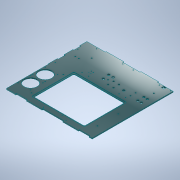
# Autodesk Inventor part: Lateral Derecho Carcasa
Saved by Autodesk Inventor 2020 (Build 240168000, 168)
## iProperties
Created: 2020-06-08
Part Number: Lateral Derecho Carcasa
Material: MDF Tablero de fibras de densidad media
Document SubType Name: Modeling
Designer: Pipi
Density: 0.8 g/cm^3
Appearance: Azul - Pintura mural - Brillante
Mass: 1380.71 g
Surface Area: 4227.94 cm^2
Volume: 1725.88 cm^3
Author: Pipi
Autodesk Inventor part; units mm, degrees
ref_plane "YZ Plane" through (0, 0, 0) normal (1, 0, 0) x (0, 1, 0)
ref_plane "XZ Plane" through (0, 0, 0) normal (0, 1, 0) x (-1, 0, 0)
ref_plane "XY Plane" through (0, 0, 0) normal (0, 0, 1) x (1, 0, 0)
sketch "Boceto1" plane through (0, 0, 0) normal (0, 1, 0) x (-1, 0, 0)
  line L0 (31.3028, -81.5323) -> (31.3028, -546.5323)
  line L1 (526.8028, -376.5323) -> (521.3028, -376.5323)
  line L2 (116.3028, -128.5323) -> (116.3028, -344.5323)
  line L3 (398.303, -351.5323) -> (123.3028, -351.5323)
  line L4 (123.3028, -121.5323) -> (399.3028, -121.5323)
  line L5 (526.8028, -376.5323) -> (526.8028, -326.5323)
  line L6 (521.3028, -416.5323) -> (521.3028, -376.5323)
  line L7 (406.3028, -344.5323) -> (406.3028, -128.5323)
  line L8 (399.3028, -351.5323) -> (123.3028, -351.5323)
  line L9 (123.3028, -121.5323) -> (399.3028, -121.5323)
  arc A0 (399.3028, -351.5323) -> (406.3028, -344.5323) centre (399.3028, -344.5323) ccw
  arc A1 (406.3028, -128.5323) -> (399.3028, -121.5323) centre (399.3028, -128.5323) ccw
  arc A2 (123.3028, -121.5323) -> (116.3028, -128.5323) centre (123.3028, -128.5323) ccw
  arc A3 (116.3028, -344.5323) -> (123.3028, -351.5323) centre (123.3028, -344.5323) ccw
  line L10 (123.3028, -114.5323) -> (399.3028, -114.5323)
  line L11 (413.3028, -128.5323) -> (413.3028, -344.5323)
  line L12 (399.3028, -358.5323) -> (123.3028, -358.5323)
  line L13 (109.3028, -344.5323) -> (109.3028, -128.5323)
  line L14 (109.3028, -128.5323) -> (109.3028, -121.5323)
  line L15 (116.3028, -114.5323) -> (123.3028, -114.5323)
  line L16 (109.3028, -344.5323) -> (109.3028, -351.5323)
  line L17 (116.3028, -358.5323) -> (123.3028, -358.5323)
  line L18 (413.3028, -344.5323) -> (413.3028, -351.5323)
  line L19 (406.3028, -358.5323) -> (399.3028, -358.5323)
  line L20 (413.3028, -128.5323) -> (413.3028, -121.5323)
  line L21 (399.3028, -114.5323) -> (406.3028, -114.5323)
  arc A4 (413.3028, -121.5323) -> (406.3028, -114.5323) centre (406.3028, -121.5323) ccw
  arc A5 (406.3028, -358.5323) -> (413.3028, -351.5323) centre (406.3028, -351.5323) ccw
  arc A6 (109.3028, -351.5323) -> (116.3028, -358.5323) centre (116.3028, -351.5323) ccw
  arc A7 (116.3028, -114.5323) -> (109.3028, -121.5323) centre (116.3028, -121.5323) ccw
  line L22 (421.3028, -552.0323) -> (421.3028, -546.5323)
  line L23 (421.3028, -546.5323) -> (521.3028, -546.5323)
  line L24 (421.3028, -552.0323) -> (321.3028, -552.0323)
  line L25 (321.3028, -552.0323) -> (321.3028, -546.5323)
  line L26 (321.3028, -546.5323) -> (221.3028, -546.5323)
  line L27 (221.3028, -546.5323) -> (221.3028, -552.0323)
  line L28 (319.3028, -81.5323) -> (319.3028, -87.0323)
  line L29 (199.3028, -81.5323) -> (199.3028, -87.0323)
  line L30 (319.3028, -87.0323) -> (199.3028, -87.0323)
  circle A8 centre (76.3028, -156.5323) radius 3
  circle A9 centre (76.3028, -276.5323) radius 3
  line L31 (31.3028, -81.5323) -> (49.3028, -81.5323)
  circle A10 centre (76.3028, -481.0323) radius 3
  line L32 (521.3028, -81.5323) -> (523.8028, -81.5323)
  line L33 (221.3028, -552.0323) -> (121.3028, -552.0323)
  line L34 (121.3028, -552.0323) -> (121.3028, -546.5323)
  line L35 (121.3028, -546.5323) -> (31.3028, -546.5323)
  line L36 (526.8028, -416.5323) -> (521.3028, -416.5323)
  line L37 (526.8028, -416.5323) -> (526.8028, -466.5323)
  line L38 (526.8028, -466.5323) -> (521.3028, -466.5323)
  line L39 (521.3028, -466.5323) -> (521.3028, -506.5323)
  line L40 (521.3028, -506.5323) -> (526.8028, -506.5323)
  line L41 (526.8028, -546.5323) -> (526.8028, -506.5323)
  circle A11 centre (41.0178, -541.5323) radius 2
  circle A12 centre (349.1778, -378.6573) radius 2
  circle A13 centre (386.4278, -378.6573) radius 2
  circle A14 centre (367.8028, -383.8623) radius 2
  line L42 (261.3028, -358.5323) -> (261.3028, -396.5323)
  circle A15 centre (173.4278, -378.6573) radius 2
  circle A16 centre (136.1778, -378.6573) radius 2
  line L43 (521.3028, -546.5323) -> (526.8028, -546.5323)
  circle A17 centre (194.3028, -94.7473) radius 2
  circle A18 centre (324.3028, -94.7473) radius 2
  circle A19 centre (461.8028, -538.0323) radius 2
  circle A20 centre (311.8028, -538.0323) radius 2
  circle A21 centre (101.3028, -538.0323) radius 2
  circle A22 centre (251.3028, -538.0323) radius 2
  circle A23 centre (513.5878, -481.5323) radius 2
  circle A24 centre (513.5878, -351.5323) radius 2
  line L44 (319.3028, -81.5323) -> (409.3028, -81.5323)
  line L45 (409.3028, -81.5323) -> (409.3028, -87.0323)
  line L46 (409.3028, -87.0323) -> (469.3028, -87.0323)
  line L47 (469.3028, -87.0323) -> (469.3028, -81.5323)
  line L48 (521.3028, -81.5323) -> (469.3028, -81.5323)
  line L49 (409.3028, -81.5323) -> (319.3028, -81.5323)
  line L50 (199.3028, -81.5323) -> (109.3028, -81.5323)
  line L51 (109.3028, -81.5323) -> (109.3028, -87.0323)
  line L52 (109.3028, -87.0323) -> (49.3028, -87.0323)
  line L53 (49.3028, -87.0323) -> (49.3028, -81.5323)
  line L54 (31.3028, -81.5323) -> (49.3028, -81.5323)
  line L55 (109.3028, -81.5323) -> (199.3028, -81.5323)
  circle A25 centre (354.4278, -397.5323) radius 1.5
  circle A26 centre (366.4278, -397.5323) radius 1.5
  line L56 (82.3528, -532.0323) -> (70.2528, -532.0323)
  line L57 (70.2528, -532.0323) -> (70.2528, -542.7823)
  line L58 (70.2528, -542.7823) -> (82.3528, -542.7823)
  line L59 (82.3528, -542.7823) -> (82.3528, -532.0323)
  line L60 (69.2528, -543.7823) -> (69.2528, -531.0323)
  line L61 (69.2528, -531.0323) -> (83.3528, -531.0323)
  line L62 (83.3528, -531.0323) -> (83.3528, -543.7823)
  line L63 (83.3528, -543.7823) -> (69.2528, -543.7823)
  circle A27 centre (518.3028, -143.5323) radius 2.25
  circle A28 centre (447.3028, -143.5323) radius 2.25
  circle A29 centre (447.3028, -298.5323) radius 2.25
  circle A30 centre (518.3028, -298.5323) radius 2.25
  circle A31 centre (518.3028, -214.5323) radius 2.25
  circle A32 centre (518.3028, -227.5323) radius 2.25
  circle A33 centre (447.3028, -214.5323) radius 2.25
  circle A34 centre (447.3028, -227.5323) radius 2.25
  circle A35 centre (482.8028, -179.0323) radius 37.5
  circle A36 centre (482.8028, -263.0323) radius 37.5
  line L64 (523.8028, -81.5323) -> (524.4028, -81.5323)
  line L65 (524.4028, -81.5323) -> (524.4028, -326.5323)
  line L66 (524.4028, -326.5323) -> (526.8028, -326.5323)
  circle A37 centre (484.8028, -438.5323) radius 3
  circle A38 centre (464.8028, -438.5323) radius 3
  circle A39 centre (366.4278, -411.5323) radius 2
  circle A40 centre (354.4278, -411.5323) radius 2
  circle A41 centre (228.4028, -106.5323) radius 2
  point P0 (0, 0)
  point P1 (398.3028, -355.6989)
  point P2 (109.3028, -358.5323)
  point P3 (413.3028, -358.5323)
  point P4 (413.3028, -114.5323)
  point P5 (398.303, -351.5323)
  dimension "d142" = 230
  dimension "d146" = 85
  dimension "d155" = 5.5
  dimension "d159" = 40
  dimension "d160" = 50
  dimension "d185" = 90
  dimension "d207" = 7
  dimension "d208" = 290
  dimension "d219" = 7
  dimension "d220" = 7
  dimension "d221" = 7
  dimension "d223" = 7
  dimension "d230" = 5.5
  dimension "d235" = 100
  dimension "d236" = 100
  dimension "d237" = 100
  dimension "d257" = 202
  dimension "d258" = 5.5
  dimension "d259" = 168
  dimension "d261" = 120
  dimension "d279" = 6
  dimension "d280" = 6
  dimension "d289" = 120
  dimension "d292" = 6
  dimension "d298" = 7
  dimension "d299" = 27.5
  dimension "d303" = 5.5
  dimension "d304" = 100
  dimension "d305" = 5.5
  dimension "d311" = 5.5
  dimension "d314" = 50
  dimension "d315" = 40
  dimension "d316" = 5.5
  dimension "d323" = 4
  dimension "d324" = 9.715
  dimension "d325" = 5
  dimension "d328" = 4
  dimension "d329" = 4
  dimension "d330" = 4
  dimension "d338" = 20.125
  dimension "d339" = 25.33
  dimension "d340" = 20.125
  dimension "d341" = 26.875
  dimension "d355" = 4
  dimension "d356" = 163
  dimension "d357" = 4
  dimension "d358" = 130
  dimension "d361" = 4
  dimension "d362" = 8.5
  dimension "d363" = 65
  dimension "d364" = 4
  dimension "d365" = 150
  dimension "d366" = 4
  dimension "d367" = 8.5
  dimension "d368" = 70
  dimension "d369" = 4
  dimension "d370" = 150
  dimension "d371" = 4
  dimension "d372" = 65
  dimension "d373" = 7.715
  dimension "d374" = 4
  dimension "d375" = 7.715
  dimension "d376" = 130
  dimension "d377" = 7.715
  constraints: 134 end point, 42 centre point, 27 perpendicular, 16 point on circle, 16 tangent, 12 horizontal, 10 point on line, 9 vertical, 6 equal radius, 5 parallel, 2 symmetric about line, 1 midpoint, 5 other
  measures "d142" distance between parallel lines of L3 L4
  measures "d146" distance between parallel lines of L0 L2
  measures "d155" distance between parallel lines of L6 L5
  measures "d159" distance of L6.start L1.end
  measures "d160" distance of L1.start L5.end
  measures "d185" angle of L1 L5
  measures "d207" radius of A0
  measures "d208" distance between parallel lines of L2 L7
  measures "d219" distance between parallel lines of L7 L11
  measures "d220" distance between parallel lines of L2 L13
  measures "d221" radius of A4
  measures "d223" distance between parallel lines of L3 L12
  measures "d230" distance of L22.start L22.end
  measures "d235" distance of L22.end L23.end
  measures "d236" distance of L22.start L24.end
  measures "d237" distance of L25.end L26.end
  measures "d257" distance of L32.start L28.start
  measures "d258" distance of L28.start L28.end
  measures "d259" distance of L0.start L29.start
  measures "d261" distance of L28.end L29.end
  measures "d279" diameter of A8
  measures "d280" diameter of A9
  measures "d289" distance of A8.centre A9.centre
  measures "d292" diameter of A10
  measures "d298" distance between parallel lines of L10 L4
  measures "d299" distance between parallel lines of L30 L10
  measures "d303" distance of L41.start L23.end
  measures "d304" distance of L27.end L33.end
  measures "d305" distance of L26.end L27.end
  measures "d311" distance of L33.end L34.end
  measures "d314" distance of L36.start L37.end
  measures "d315" distance of L38.end L39.end
  measures "d316" distance of L39.end L40.end
  measures "d323" diameter of A11
  measures "d324" distance from line of L0 A11.centre
  measures "d325" distance from line of L35 A11.centre
  measures "d328" diameter of A12
  measures "d329" diameter of A13
  measures "d330" diameter of A14
  measures "d338" distance from line of L12 A13.centre
  measures "d339" distance from line of L12 A14.centre
  measures "d340" distance from line of L12 A12.centre
  measures "d341" distance from line of L18 A13.centre
  measures "d355" diameter of A17
  measures "d356" distance from line of L0 A17.centre
  measures "d357" diameter of A18
  measures "d358" distance of A17.centre A18.centre
  measures "d361" diameter of A19
  measures "d362" distance from line of L23 A19.centre
  measures "d363" distance from line of L41 A19.centre
  measures "d364" diameter of A20
  measures "d365" distance of A20.centre A19.centre
  measures "d366" diameter of A21
  measures "d367" distance from line of L35 A21.centre
  measures "d368" distance from line of L0 A21.centre
  measures "d369" diameter of A22
  measures "d370" distance of A21.centre A22.centre
  measures "d371" diameter of A23
  measures "d372" distance from line of L23 A23.centre
  measures "d373" distance from line of L39 A23.centre
  measures "d374" diameter of A24
  measures "d375" distance from line of L6 A24.centre
  measures "d376" distance of A23.centre A24.centre
  measures "d377" distance from line of A18.centre L30
extrude "Extrusión1" add sketch "Boceto1" along normal blind 5.5 contours L31 L53 L52 L51 L50 L29 L30 L28 L44 L45 L46 L47 L48 L32 L64 L65 L66 L5 L1 L6 L36 L37 L38 L39 L40 L41 L43 L23 L22 L24 L25 L26 L27 L33 L34 L35 L0 | A14
extrude "Extrusión3" add sketch "Boceto1" along normal blind 2.5 contours L10 L21 A4 L20 L11 L18 A5 L19 L12 L17 A6 L16 L13 L14 A7 L15
sketch "Boceto2" plane through (0, 0, 0) normal (0, -1, 0) x (1, 0, 0)
  line L0 (-31.3028, -81.5323) -> (-31.3028, -546.5323) projected
  line L1 (-51.3028, -384.3323) -> (-51.3028, -448.8323)
  line L2 (-233.4894, -384.3323) -> (-51.3028, -384.3323)
  line L3 (-233.4894, -384.3323) -> (-310.8028, -384.3323)
  line L4 (-51.3028, -384.3323) -> (-51.3028, -448.8323)
  line L5 (-51.3028, -448.8323) -> (-310.8028, -448.8323)
  line L6 (-310.8028, -448.8323) -> (-310.8028, -384.3323)
  line L7 (-51.3028, -384.3323) -> (-51.3028, -409.3323)
  circle A0 centre (-177.3028, -408.8323) radius 6
  circle A1 centre (-294.3028, -408.8323) radius 6
  line L8 (-256.8028, -429.8323) -> (-256.8028, -387.8323)
  line L9 (-256.8028, -387.8323) -> (-214.8028, -387.8323)
  line L10 (-256.8028, -429.8323) -> (-214.8028, -429.8323)
  line L11 (-214.8028, -429.8323) -> (-214.8028, -387.8323)
  line L12 (-256.8028, -429.8323) -> (-256.8028, -424.3323)
  line L13 (-220.3028, -424.3323) -> (-220.3028, -393.3323)
  line L14 (-214.8028, -387.8323) -> (-214.8028, -393.3323)
  line L15 (-220.3028, -393.3323) -> (-251.3028, -393.3323)
  line L16 (-251.3028, -424.3323) -> (-251.3028, -393.3323)
  line L17 (-251.3028, -424.3323) -> (-220.3028, -424.3323)
  circle A2 centre (-251.3028, -424.3323) radius 4
  circle A3 centre (-251.3028, -393.3323) radius 4
  circle A4 centre (-220.3028, -424.3323) radius 4
  circle A5 centre (-220.3028, -393.3323) radius 4
  line L18 (-310.8028, -448.8323) -> (-310.8028, -443.8323)
  line L19 (-310.8028, -443.8323) -> (-298.3028, -443.8323)
  line L20 (-298.3028, -443.8323) -> (-273.3028, -443.8323)
  circle A6 centre (-298.3028, -443.8323) radius 6
  circle A7 centre (-273.3028, -443.8323) radius 6
  circle A8 centre (-66.3028, -433.8323) radius 6
  circle A9 centre (-86.3028, -433.8323) radius 6
  circle A10 centre (-86.3028, -398.8323) radius 6
  circle A11 centre (-66.3028, -398.8323) radius 6
  line L21 (-235.8028, -429.8323) -> (-235.8028, -387.8323)
  line L22 (-256.8028, -408.8323) -> (-214.8028, -408.8323)
  line L23 (-399.3028, -351.5323) -> (-123.3028, -351.5323) projected
  circle A12 centre (-131.3028, -430.8323) radius 3
  circle A13 centre (-131.3028, -402.3323) radius 3
  circle A14 centre (-275.8028, -416.8323) radius 3
  line L24 (-51.3028, -448.8323) -> (-310.8028, -448.8323)
  line L25 (-310.8028, -448.8323) -> (-310.8028, -384.3323)
  line L26 (-310.8028, -448.8323) -> (-310.8028, -443.8323)
  line L27 (-310.8028, -443.8323) -> (-298.3028, -443.8323)
  line L28 (-298.3028, -443.8323) -> (-273.3028, -443.8323)
  circle A15 centre (-298.3028, -443.8323) radius 6
  circle A16 centre (-273.3028, -443.8323) radius 6
  line L29 (-51.3028, -448.8323) -> (-310.8028, -448.8323)
  line L30 (-310.8028, -448.8323) -> (-310.8028, -384.3323)
  line L31 (-310.8028, -448.8323) -> (-310.8028, -443.8323)
  line L32 (-310.8028, -443.8323) -> (-298.3028, -443.8323)
  line L33 (-298.3028, -443.8323) -> (-273.3028, -443.8323)
  circle A17 centre (-298.3028, -443.8323) radius 6
  circle A18 centre (-273.3028, -443.8323) radius 6
  line L34 (-51.3028, -448.8323) -> (-310.8028, -448.8323)
  line L35 (-310.8028, -448.8323) -> (-310.8028, -384.3323)
  line L36 (-310.8028, -448.8323) -> (-310.8028, -443.8323)
  line L37 (-310.8028, -443.8323) -> (-298.3028, -443.8323)
  line L38 (-298.3028, -443.8323) -> (-273.3028, -443.8323)
  circle A19 centre (-298.3028, -443.8323) radius 6
  circle A20 centre (-273.3028, -443.8323) radius 6
  line L39 (-51.3028, -448.8323) -> (-310.8028, -448.8323)
  line L40 (-310.8028, -448.8323) -> (-310.8028, -384.3323)
  line L41 (-310.8028, -448.8323) -> (-310.8028, -443.8323)
  line L42 (-310.8028, -443.8323) -> (-298.3028, -443.8323)
  line L43 (-298.3028, -443.8323) -> (-273.3028, -443.8323)
  circle A21 centre (-298.3028, -443.8323) radius 6
  circle A22 centre (-273.3028, -443.8323) radius 6
  line L44 (-51.3028, -448.8323) -> (-310.8028, -448.8323)
  line L45 (-310.8028, -448.8323) -> (-310.8028, -384.3323)
  line L46 (-310.8028, -448.8323) -> (-310.8028, -443.8323)
  line L47 (-310.8028, -443.8323) -> (-298.3028, -443.8323)
  line L48 (-298.3028, -443.8323) -> (-273.3028, -443.8323)
  circle A23 centre (-298.3028, -443.8323) radius 6
  circle A24 centre (-273.3028, -443.8323) radius 6
  line L49 (-51.3028, -448.8323) -> (-310.8028, -448.8323)
  line L50 (-310.8028, -448.8323) -> (-310.8028, -384.3323)
  line L51 (-310.8028, -448.8323) -> (-310.8028, -443.8323)
  line L52 (-310.8028, -443.8323) -> (-298.3028, -443.8323)
  line L53 (-298.3028, -443.8323) -> (-273.3028, -443.8323)
  circle A25 centre (-298.3028, -443.8323) radius 6
  circle A26 centre (-273.3028, -443.8323) radius 6
  line L54 (-51.3028, -448.8323) -> (-310.8028, -448.8323)
  line L55 (-310.8028, -448.8323) -> (-310.8028, -384.3323)
  line L56 (-310.8028, -448.8323) -> (-310.8028, -443.8323)
  line L57 (-310.8028, -443.8323) -> (-298.3028, -443.8323)
  line L58 (-298.3028, -443.8323) -> (-273.3028, -443.8323)
  circle A27 centre (-298.3028, -443.8323) radius 6
  circle A28 centre (-273.3028, -443.8323) radius 6
  line L59 (-51.3028, -448.8323) -> (-310.8028, -448.8323)
  line L60 (-310.8028, -448.8323) -> (-310.8028, -384.3323)
  line L61 (-310.8028, -448.8323) -> (-310.8028, -443.8323)
  line L62 (-310.8028, -443.8323) -> (-298.3028, -443.8323)
  line L63 (-298.3028, -443.8323) -> (-273.3028, -443.8323)
  circle A29 centre (-298.3028, -443.8323) radius 6
  circle A30 centre (-273.3028, -443.8323) radius 6
  point P0 (0, 0)
  point P1 (-31.3028, -85.6989)
  point P2 (-521.3028, -627.1989)
  point P3 (-31.3028, -532.1989)
  dimension "d68" = 64.5
  dimension "d69" = 259.5
  dimension "d70" = 20
  dimension "d71" = 25
  dimension "d73" = 12
  dimension "d75" = 12
  dimension "d76" = 126
  dimension "d77" = 243
  dimension "d78" = 42
  dimension "d79" = 42
  dimension "d80" = 5.5
  dimension "d82" = 5.5
  dimension "d83" = 5.5
  dimension "d84" = 8
  dimension "d85" = 8
  dimension "d86" = 8
  dimension "d87" = 8
  dimension "d88" = 3.5
  dimension "d91" = 5
  dimension "d92" = 12.5
  dimension "d93" = 25
  dimension "d94" = 12
  dimension "d95" = 12
  dimension "d96" = 12
  dimension "d97" = 12
  dimension "d98" = 12
  dimension "d99" = 12
  dimension "d102" = 20
  dimension "d103" = 15
  dimension "d106" = 20
  dimension "d107" = 15
  dimension "d148" = 58.5
  dimension "d193" = 5.5
  dimension "d194" = 5.5
  dimension "d213" = 35
  dimension "d214" = 35
  dimension "d263" = 6
  dimension "d264" = 6
  dimension "d269" = 6
  dimension "d273" = 18
  dimension "d274" = 18
  dimension "d275" = 32
  dimension "d300" = 90
  dimension "d301" = 32.8
  dimension "d383" = 40
  dimension "d384" = 40
  dimension "d385" = 15
  dimension "d386" = 15
  dimension "d457" = 259.5
  dimension "d458" = 5
  dimension "d459" = 12.5
  dimension "d460" = 25
  dimension "d461" = 12
  dimension "d462" = 12
  dimension "d463" = 259.5
  dimension "d464" = 5
  dimension "d465" = 12.5
  dimension "d466" = 25
  dimension "d467" = 12
  dimension "d468" = 12
  dimension "d469" = 259.5
  dimension "d470" = 5
  dimension "d471" = 12.5
  dimension "d472" = 25
  constraints: 124 end point, 31 centre point, 22 coincident, 21 point on line, 17 perpendicular, 4 midpoint, 2 horizontal, 2 vertical
  measures "d68" distance of L1.end L1.start
  measures "d69" distance of L1.end L5.end
  measures "d70" distance between parallel lines of L0 L1
  measures "d71" distance of L1.start L7.end
  measures "d73" diameter of A0
  measures "d75" diameter of A1
  measures "d76" distance from line of L7 A0.centre
  measures "d77" distance from line of A1.centre L1
  measures "d78" distance of L8.start L8.end
  measures "d79" distance of L8.end L9.end
  measures "d80" distance of L8.start L12.end
  measures "d82" distance of L9.end L14.end
  measures "d83" distance of L16.start L12.end
  measures "d84" diameter of A2
  measures "d85" diameter of A3
  measures "d86" diameter of A4
  measures "d87" diameter of A5
  measures "d88" distance between parallel lines of L3 L9
  measures "d91" distance of L5.end L18.end
  measures "d92" distance of L18.end L19.end
  measures "d93" distance of L19.end L20.end
  measures "d94" diameter of A6
  measures "d95" diameter of A7
  measures "d96" diameter of A8
  measures "d97" diameter of A9
  measures "d98" diameter of A10
  measures "d99" diameter of A11
  measures "d102" distance of A9.centre A8.centre
  measures "d103" distance from line of L1 A8.centre
  measures "d106" distance of A11.centre A10.centre
  measures "d107" distance from line of L7 A11.centre
  measures "d148" distance from line of A0.centre L21
  measures "d193" distance between parallel lines of L9 L15
  measures "d194" distance between parallel lines of L10 L17
  measures "d213" distance of A11.centre A8.centre
  measures "d214" distance of A10.centre A9.centre
  measures "d263" diameter of A12
  measures "d264" diameter of A13
  measures "d269" diameter of A14
  measures "d273" distance from line of L5 A12.centre
  measures "d274" distance from line of L2 A13.centre
  measures "d275" distance from line of L5 A14.centre
  measures "d300" angle of L2 L1
  measures "d301" distance between parallel lines of L23 L2
  measures "d383" distance from line of L5 A1.centre
  measures "d384" distance from line of L5 A0.centre
  measures "d385" distance from line of L5 A9.centre
  measures "d386" distance from line of L5 A8.centre
  measures "d457" distance of L24.start L24.end
  measures "d458" distance of L24.end L26.end
  measures "d459" distance of L26.end L28.start
  measures "d460" distance of L28.start L28.end
  measures "d461" diameter of A15
  measures "d462" diameter of A16
  measures "d463" distance of L29.start L29.end
  measures "d464" distance of L29.end L31.end
  measures "d465" distance of L31.end L33.start
  measures "d466" distance of L33.start L33.end
  measures "d467" diameter of A17
  measures "d468" diameter of A18
  measures "d469" distance of L34.start L34.end
  measures "d470" distance of L34.end L36.end
  measures "d471" distance of L36.end L38.start
  measures "d472" distance of L38.start L38.end
sketch "Boceto3" plane through (0, 5.5, 0) normal (0, 1, 0) x (1, 0, 0)
  circle A0 centre (-429.9448, 131.5323) radius 3
  circle A1 centre (-429.9448, 314.5323) radius 3
  circle A2 centre (-429.9448, 477.5323) radius 3
  line L0 (-521.3028, 506.5323) -> (-521.3028, 466.5323) projected
  line L1 (-524.4028, 326.5323) -> (-524.4028, 81.5323) projected
  line L2 (-524.4028, 81.5323) -> (-469.3028, 81.5323) projected
  line L3 (-526.8028, 466.5323) -> (-526.8028, 416.5323) projected
  point P0 (0, 0)
  point P1 (-319.3028, 81.5323)
  point P2 (-524.4028, 81.5323)
  dimension "d167" = 6
  dimension "d168" = 6
  dimension "d169" = 6
  dimension "d318" = 183
  dimension "d319" = 163
  dimension "d441" = 94.458
  dimension "d442" = 94.458
  dimension "d445" = 50
  dimension "d456" = 94.458
  constraints: 3 centre point
  measures "d167" diameter of A0
  measures "d168" diameter of A1
  measures "d169" diameter of A2
  measures "d318" distance of A1.centre A0.centre
  measures "d319" distance of A2.centre A1.centre
  measures "d441" distance from line of L1 A0.centre
  measures "d442" distance from line of L1 A1.centre
  measures "d445" distance from line of L2 A0.centre
  measures "d456" distance from line of A2.centre L1
extrude "Extrusión5" cut sketch "Boceto3" against normal blind 10
extrude "Extrusión6" cut sketch "Boceto2" against normal blind 10 contours A7 L5 | L5 A7 | A6 L20 L19 | L19 L20 A6 L5 | A6 L5 | A0 | A1 | A2 L16 L17 | L17 L16 A2 | A4 L13 L17 | L17 L13 A4 | A3 L15 L16 | L16 L15 A3 | A5 L15 L13 | L13 L15 A5 | A8 | A9 | A10 | A11 | A12 | A13 | A14
